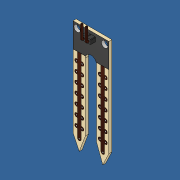
# Autodesk Inventor part: Soil-Moisture-Sensor-Probe
Saved by Autodesk Inventor 2018 (Build 220112000, 112)
## iProperties
Created: 2017-12-22
Part Number: Soil-Moisture-Sensor-Probe
Material: Generisch
Document SubType Name: Modeling
Designer: Martin
Density: 1 g/cm^3
Appearance: Vorgabe
Author: Martin
Autodesk Inventor part; units mm, degrees
ref_plane "YZ Plane" through (0, 0, 0) normal (1, 0, 0) x (0, 1, 0)
sketch "Skizze1" plane through (0, 0, 0) normal (0, 1, 0) x (-1, 0, 0)
  line L0 (9.75, 0) -> (9.75, -53)
  line L1 (9.75, -53) -> (6.4, -60)
  line L2 (6.4, -60) -> (3.05, -51)
  line L3 (3.05, -51) -> (3.05, -14.35)
  arc A0 (3.05, -14.35) -> (-3.05, -14.35) centre (0, -14.35) ccw
  line L4 (-3.05, -14.35) -> (-3.05, -51)
  line L5 (-3.05, -51) -> (-6.4, -60)
  line L6 (-6.4, -60) -> (-9.75, -53)
  line L7 (-9.75, -53) -> (-9.75, 0)
  line L8 (-9.75, 0) -> (9.75, 0)
  line L9 (6.4, -60) -> (-6.4, -60) construction
  line L10 (0, -60) -> (0, -14.35) construction
  circle A1 centre (7.5, -2.5) radius 1.75
  circle A2 centre (-7.5, -2.5) radius 1.75
  line L11 (7.5, -2.5) -> (-7.5, -2.5) construction
  line L12 (0, -2.5) -> (0, -14.35) construction
  point P0 (0, 0)
  point P1 (0, 0)
  dimension "d0" = 19.5
  dimension "d1" = 60
  dimension "d2" = 6.7
  dimension "d3" = 6.7
  dimension "d4" = 11.3
  dimension "d5" = 7
  dimension "d6" = 9
  dimension "d7" = 12.8
  dimension "d8" = 15
  dimension "d9" = 3.5
  dimension "d10" = 0.75
  constraints: 26 end point, 3 centre point, 3 midpoint, 3 parallel, 3 vertical, 2 equal length, 2 horizontal, 2 point on circle, 2 tangent, 1 coincident, 1 equal radius, 1 perpendicular
  measures "d0" distance between parallel lines of L7 L0
  measures "d1" distance from line of L5.end L8
  measures "d2" distance between parallel lines of L7 L4
  measures "d3" distance between parallel lines of L0 L3
  measures "d4" distance edge to line of A0 L8
  measures "d5" vertical distance of L5.end L6.end
  measures "d6" vertical distance of L4.end L5.end
  measures "d7" distance of L1.end L5.end
  measures "d8" distance of L11.start L11.end
  measures "d9" diameter of A2
  measures "d10" distance edge to line of A2 L8
extrude "Extrusion1" add sketch "Skizze1" against normal blind 1.6
sketch "Skizze2" plane through (0, -1.6, 0) normal (0, -1, 0) x (1, 0, 0)
  circle A0 centre (7.5, -2.5) radius 1.75 projected
  circle A1 centre (-7.5, -2.5) radius 1.75 projected
  line L0 (-9.75, 0) -> (-9.75, -53) projected
  line L1 (-9.75, -53) -> (-6.4, -60) projected
  line L2 (-6.4, -60) -> (-3.05, -51) projected
  line L3 (-3.05, -51) -> (-3.05, -14.35) projected
  arc A2 (3.05, -14.35) -> (-3.05, -14.35) centre (0, -14.35) ccw projected
  line L4 (3.05, -14.35) -> (3.05, -51) projected
  line L5 (3.05, -51) -> (6.4, -60) projected
  line L6 (6.4, -60) -> (9.75, -53) projected
  line L7 (9.75, -53) -> (9.75, 0) projected
  line L8 (9.75, 0) -> (-9.75, 0) projected
  line L9 (-7.4, -13.3) -> (-5.4, -13.3)
  line L10 (-5.4, -13.3) -> (-5.4, -54)
  line L11 (-6.4, -55) -> (-6.4, -55)
  line L12 (-7.4, -54) -> (-7.4, -13.3)
  line L13 (5.4, -13.3) -> (7.4, -13.3)
  line L14 (7.4, -13.3) -> (7.4, -54)
  line L15 (6.4, -55) -> (6.4, -55)
  line L16 (5.4, -54) -> (5.4, -13.3)
  arc A3 (5.4, -54) -> (6.4, -55) centre (6.4, -54) ccw
  arc A4 (6.4, -55) -> (7.4, -54) centre (6.4, -54) ccw
  arc A5 (-6.4, -55) -> (-5.4, -54) centre (-6.4, -54) ccw
  arc A6 (-7.4, -54) -> (-6.4, -55) centre (-6.4, -54) ccw
  point P0 (0, 0)
  dimension "d13" = 2
  dimension "d14" = 55
  dimension "d15" = 6.7
  dimension "d16" = 2.35
  dimension "d17" = 2.35
  dimension "d18" = 1
  dimension "d19" = 13.3
  constraints: 16 end point, 8 point on circle, 8 tangent, 4 centre point, 4 parallel, 3 equal radius, 2 collinear, 2 horizontal, 2 perpendicular, 1 point on line
  measures "d13" distance between parallel lines of L14 L16
  measures "d14" distance between parallel lines of L8 L15
  measures "d15" distance between parallel lines of L7 L4
  measures "d16" distance between parallel lines of L7 L14
  measures "d17" distance between parallel lines of L0 L12
  measures "d18" radius of A3
  measures "d19" distance between parallel lines of L8 L13
extrude "Extrusion2" add sketch "Skizze2" along normal blind 0.01 contours L9 L10 A5 A6 L12 | L13 L14 A4 A3 L16
sketch "Skizze3" plane through (0, -1.61, 0) normal (0, -1, 0) x (1, 0, 0)
  line L0 (-5.4, -13.3) -> (-7.4, -13.3) projected
  line L1 (-7.4, -13.3) -> (-7.4, -54) projected
  arc A0 (-7.4, -54) -> (-5.4, -54) centre (-6.4, -54) ccw projected
  line L2 (-5.4, -54) -> (-5.4, -13.3) projected
  line L3 (-8.9, -18) -> (-3.9, -18) construction
  line L4 (-7.9, -19) -> (-4.9, -19)
  line L5 (-4.9, -17) -> (-7.9, -17)
  arc A1 (-7.9, -17) -> (-7.9, -19) centre (-7.9, -18) ccw
  arc A2 (-4.9, -19) -> (-4.9, -17) centre (-4.9, -18) ccw
  line L6 (-6.4, -13.3) -> (-6.4, -54) construction
  line L7 (7.4, -13.3) -> (5.4, -13.3) construction
  arc A3 (-7.9, -22.1) -> (-7.9, -24.1) centre (-7.9, -23.1) ccw
  arc A4 (-4.9, -24.1) -> (-4.9, -22.1) centre (-4.9, -23.1) ccw
  line L8 (-7.9, -24.1) -> (-4.9, -24.1)
  line L9 (-8.9, -23.1) -> (-3.9, -23.1) construction
  line L10 (-4.9, -22.1) -> (-7.9, -22.1)
  arc A5 (-7.9, -27.2) -> (-7.9, -29.2) centre (-7.9, -28.2) ccw
  arc A6 (-4.9, -29.2) -> (-4.9, -27.2) centre (-4.9, -28.2) ccw
  line L11 (-7.9, -29.2) -> (-4.9, -29.2)
  line L12 (-8.9, -28.2) -> (-3.9, -28.2) construction
  line L13 (-4.9, -27.2) -> (-7.9, -27.2)
  arc A7 (-7.9, -32.3) -> (-7.9, -34.3) centre (-7.9, -33.3) ccw
  arc A8 (-4.9, -34.3) -> (-4.9, -32.3) centre (-4.9, -33.3) ccw
  line L14 (-7.9, -34.3) -> (-4.9, -34.3)
  line L15 (-8.9, -33.3) -> (-3.9, -33.3) construction
  line L16 (-4.9, -32.3) -> (-7.9, -32.3)
  arc A9 (-7.9, -37.4) -> (-7.9, -39.4) centre (-7.9, -38.4) ccw
  arc A10 (-4.9, -39.4) -> (-4.9, -37.4) centre (-4.9, -38.4) ccw
  line L17 (-7.9, -39.4) -> (-4.9, -39.4)
  line L18 (-8.9, -38.4) -> (-3.9, -38.4) construction
  line L19 (-4.9, -37.4) -> (-7.9, -37.4)
  arc A11 (-7.9, -42.5) -> (-7.9, -44.5) centre (-7.9, -43.5) ccw
  arc A12 (-4.9, -44.5) -> (-4.9, -42.5) centre (-4.9, -43.5) ccw
  line L20 (-7.9, -44.5) -> (-4.9, -44.5)
  line L21 (-8.9, -43.5) -> (-3.9, -43.5) construction
  line L22 (-4.9, -42.5) -> (-7.9, -42.5)
  arc A13 (-7.9, -47.6) -> (-7.9, -49.6) centre (-7.9, -48.6) ccw
  arc A14 (-4.9, -49.6) -> (-4.9, -47.6) centre (-4.9, -48.6) ccw
  line L23 (-7.9, -49.6) -> (-4.9, -49.6)
  line L24 (-8.9, -48.6) -> (-3.9, -48.6) construction
  line L25 (-4.9, -47.6) -> (-7.9, -47.6)
  arc A15 (4.9, -17) -> (4.9, -19) centre (4.9, -18) ccw
  arc A16 (7.9, -19) -> (7.9, -17) centre (7.9, -18) ccw
  line L26 (4.9, -19) -> (7.9, -19)
  line L27 (3.9, -18) -> (8.9, -18) construction
  line L28 (7.9, -17) -> (4.9, -17)
  arc A17 (4.9, -22.1) -> (4.9, -24.1) centre (4.9, -23.1) ccw
  arc A18 (7.9, -24.1) -> (7.9, -22.1) centre (7.9, -23.1) ccw
  line L29 (4.9, -24.1) -> (7.9, -24.1)
  line L30 (3.9, -23.1) -> (8.9, -23.1) construction
  line L31 (7.9, -22.1) -> (4.9, -22.1)
  arc A19 (4.9, -27.2) -> (4.9, -29.2) centre (4.9, -28.2) ccw
  arc A20 (7.9, -29.2) -> (7.9, -27.2) centre (7.9, -28.2) ccw
  line L32 (4.9, -29.2) -> (7.9, -29.2)
  line L33 (3.9, -28.2) -> (8.9, -28.2) construction
  line L34 (7.9, -27.2) -> (4.9, -27.2)
  arc A21 (4.9, -32.3) -> (4.9, -34.3) centre (4.9, -33.3) ccw
  arc A22 (7.9, -34.3) -> (7.9, -32.3) centre (7.9, -33.3) ccw
  line L35 (4.9, -34.3) -> (7.9, -34.3)
  line L36 (3.9, -33.3) -> (8.9, -33.3) construction
  line L37 (7.9, -32.3) -> (4.9, -32.3)
  arc A23 (4.9, -37.4) -> (4.9, -39.4) centre (4.9, -38.4) ccw
  arc A24 (7.9, -39.4) -> (7.9, -37.4) centre (7.9, -38.4) ccw
  line L38 (4.9, -39.4) -> (7.9, -39.4)
  line L39 (3.9, -38.4) -> (8.9, -38.4) construction
  line L40 (7.9, -37.4) -> (4.9, -37.4)
  arc A25 (4.9, -42.5) -> (4.9, -44.5) centre (4.9, -43.5) ccw
  arc A26 (7.9, -44.5) -> (7.9, -42.5) centre (7.9, -43.5) ccw
  line L41 (4.9, -44.5) -> (7.9, -44.5)
  line L42 (3.9, -43.5) -> (8.9, -43.5) construction
  line L43 (7.9, -42.5) -> (4.9, -42.5)
  arc A27 (4.9, -47.6) -> (4.9, -49.6) centre (4.9, -48.6) ccw
  arc A28 (7.9, -49.6) -> (7.9, -47.6) centre (7.9, -48.6) ccw
  line L44 (4.9, -49.6) -> (7.9, -49.6)
  line L45 (3.9, -48.6) -> (8.9, -48.6) construction
  line L46 (7.9, -47.6) -> (4.9, -47.6)
  point P0 (0, 0)
  point P1 (-6.4, -18)
  point P2 (-6.4, -23.1)
  point P3 (-6.4, -28.2)
  point P4 (-6.4, -33.3)
  point P5 (-6.4, -38.4)
  point P6 (-6.4, -43.5)
  point P7 (-6.4, -48.6)
  point P8 (6.4, -18)
  point P9 (6.4, -23.1)
  point P10 (6.4, -28.2)
  point P11 (6.4, -33.3)
  point P12 (6.4, -38.4)
  point P13 (6.4, -43.5)
  point P14 (6.4, -48.6)
  dimension "d22" = 18
  dimension "d23" = 12.8
  dimension "d24" = 3
  dimension "d25" = 2
  dimension "d28" = 5.1
  dimension "d31" = 12.8
  constraints: 114 end point, 84 point on circle, 29 point on line, 28 centre point, 4 tangent, 2 midpoint, 2 vertical, 1 horizontal, 1 parallel, 1 perpendicular, 182 other
  measures "d22" distance from line of point (0, 0) L3
  measures "d23" distance of L7.end L0.end
  measures "d24" distance of A1.centre A2.centre
  measures "d25" distance between parallel lines of L5 L4
  measures "d28" distance of A1.centre A3.centre
  measures "d31" distance of A1.centre A15.centre
extrude "Extrusion3" add sketch "Skizze3" against normal blind 0.01 contours L5 A2 L4 L2 | L2 L4 L1 L5 | L1 L4 A1 L5 | L10 A4 L8 L2 | L2 L8 L1 L10 | L1 L8 A3 L10 | L13 A6 L11 L2 | L2 L11 L1 L13 | L1 L11 A5 L13 | L16 A8 L14 L2 | L2 L14 L1 L16 | L1 L14 A7 L16 | L19 A10 L17 L2 | L2 L17 L1 L19 | L1 L17 A9 L19 | L22 A12 L20 L2 | L2 L20 L1 L22 | L1 L20 A11 L22 | L25 A14 L23 L2 | L2 L23 L1 L25 | L1 L23 A13 L25 | L28 A16 L26 A15 | L31 A18 L29 A17 | L34 A20 L32 A19 | L37 A22 L35 A21 | L40 A24 L38 A23 | L43 A26 L41 A25 | L46 A28 L44 A27
ref_plane "Arbeitsebene1" through (0, -0.8, 0) normal (0, -1, 0) x (1, 0, 0)
sketch "Skizze4" plane through (0, -1.6, 0) normal (0, -1, 0) x (1, 0, 0)
  line L0 (-4.9, -49.6) -> (-5.4, -49.6) projected
  line L1 (-5.4, -49.6) -> (-5.4, -54) projected
  arc A0 (-7.4, -54) -> (-5.4, -54) centre (-6.4, -54) ccw projected
  line L2 (-7.4, -54) -> (-7.4, -49.6) projected
  line L3 (-7.4, -49.6) -> (-7.9, -49.6) projected
  arc A1 (-7.9, -47.6) -> (-7.9, -49.6) centre (-7.9, -48.6) ccw projected
  line L4 (-7.9, -47.6) -> (-7.4, -47.6) projected
  line L5 (-7.4, -47.6) -> (-7.4, -44.5) projected
  line L6 (-7.4, -44.5) -> (-7.9, -44.5) projected
  arc A2 (-7.9, -42.5) -> (-7.9, -44.5) centre (-7.9, -43.5) ccw projected
  line L7 (-7.9, -42.5) -> (-7.4, -42.5) projected
  line L8 (-7.4, -42.5) -> (-7.4, -39.4) projected
  line L9 (-7.4, -39.4) -> (-7.9, -39.4) projected
  arc A3 (-7.9, -37.4) -> (-7.9, -39.4) centre (-7.9, -38.4) ccw projected
  line L10 (-7.9, -37.4) -> (-7.4, -37.4) projected
  line L11 (-7.4, -37.4) -> (-7.4, -34.3) projected
  line L12 (-7.4, -34.3) -> (-7.9, -34.3) projected
  arc A4 (-7.9, -32.3) -> (-7.9, -34.3) centre (-7.9, -33.3) ccw projected
  line L13 (-7.9, -32.3) -> (-7.4, -32.3) projected
  line L14 (-7.4, -32.3) -> (-7.4, -29.2) projected
  line L15 (-7.4, -29.2) -> (-7.9, -29.2) projected
  arc A5 (-7.9, -27.2) -> (-7.9, -29.2) centre (-7.9, -28.2) ccw projected
  line L16 (-7.9, -27.2) -> (-7.4, -27.2) projected
  line L17 (-7.4, -27.2) -> (-7.4, -24.1) projected
  line L18 (-7.4, -24.1) -> (-7.9, -24.1) projected
  arc A6 (-7.9, -22.1) -> (-7.9, -24.1) centre (-7.9, -23.1) ccw projected
  line L19 (-7.9, -22.1) -> (-7.4, -22.1) projected
  line L20 (-7.4, -22.1) -> (-7.4, -19) projected
  line L21 (-7.4, -19) -> (-7.9, -19) projected
  arc A7 (-7.9, -17) -> (-7.9, -19) centre (-7.9, -18) ccw projected
  line L22 (-7.9, -17) -> (-7.4, -17) projected
  line L23 (-7.4, -17) -> (-7.4, -13.3) projected
  line L24 (-7.4, -13.3) -> (-5.4, -13.3) projected
  line L25 (-5.4, -13.3) -> (-5.4, -17) projected
  line L26 (-5.4, -17) -> (-4.9, -17) projected
  arc A8 (-4.9, -19) -> (-4.9, -17) centre (-4.9, -18) ccw projected
  line L27 (-4.9, -19) -> (-5.4, -19) projected
  line L28 (-5.4, -19) -> (-5.4, -22.1) projected
  line L29 (-5.4, -22.1) -> (-4.9, -22.1) projected
  arc A9 (-4.9, -24.1) -> (-4.9, -22.1) centre (-4.9, -23.1) ccw projected
  line L30 (-4.9, -24.1) -> (-5.4, -24.1) projected
  line L31 (-5.4, -24.1) -> (-5.4, -27.2) projected
  line L32 (-5.4, -27.2) -> (-4.9, -27.2) projected
  arc A10 (-4.9, -29.2) -> (-4.9, -27.2) centre (-4.9, -28.2) ccw projected
  line L33 (-4.9, -29.2) -> (-5.4, -29.2) projected
  line L34 (-5.4, -29.2) -> (-5.4, -32.3) projected
  line L35 (-5.4, -32.3) -> (-4.9, -32.3) projected
  arc A11 (-4.9, -34.3) -> (-4.9, -32.3) centre (-4.9, -33.3) ccw projected
  line L36 (-4.9, -34.3) -> (-5.4, -34.3) projected
  line L37 (-5.4, -34.3) -> (-5.4, -37.4) projected
  line L38 (-5.4, -37.4) -> (-4.9, -37.4) projected
  arc A12 (-4.9, -39.4) -> (-4.9, -37.4) centre (-4.9, -38.4) ccw projected
  line L39 (-4.9, -39.4) -> (-5.4, -39.4) projected
  line L40 (-5.4, -39.4) -> (-5.4, -42.5) projected
  line L41 (-5.4, -42.5) -> (-4.9, -42.5) projected
  arc A13 (-4.9, -44.5) -> (-4.9, -42.5) centre (-4.9, -43.5) ccw projected
  line L42 (-4.9, -44.5) -> (-5.4, -44.5) projected
  line L43 (-5.4, -44.5) -> (-5.4, -47.6) projected
  line L44 (-5.4, -47.6) -> (-4.9, -47.6) projected
  arc A14 (-4.9, -49.6) -> (-4.9, -47.6) centre (-4.9, -48.6) ccw projected
  line L45 (7.9, -44.5) -> (7.4, -44.5) projected
  line L46 (7.4, -44.5) -> (7.4, -47.6) projected
  line L47 (7.4, -47.6) -> (7.9, -47.6) projected
  arc A15 (7.9, -49.6) -> (7.9, -47.6) centre (7.9, -48.6) ccw projected
  line L48 (7.9, -49.6) -> (7.4, -49.6) projected
  line L49 (7.4, -49.6) -> (7.4, -54) projected
  arc A16 (5.4, -54) -> (7.4, -54) centre (6.4, -54) ccw projected
  line L50 (5.4, -54) -> (5.4, -49.6) projected
  line L51 (5.4, -49.6) -> (4.9, -49.6) projected
  arc A17 (4.9, -47.6) -> (4.9, -49.6) centre (4.9, -48.6) ccw projected
  line L52 (4.9, -47.6) -> (5.4, -47.6) projected
  line L53 (5.4, -47.6) -> (5.4, -44.5) projected
  line L54 (5.4, -44.5) -> (4.9, -44.5) projected
  arc A18 (4.9, -42.5) -> (4.9, -44.5) centre (4.9, -43.5) ccw projected
  line L55 (4.9, -42.5) -> (5.4, -42.5) projected
  line L56 (5.4, -42.5) -> (5.4, -39.4) projected
  line L57 (5.4, -39.4) -> (4.9, -39.4) projected
  arc A19 (4.9, -37.4) -> (4.9, -39.4) centre (4.9, -38.4) ccw projected
  line L58 (4.9, -37.4) -> (5.4, -37.4) projected
  line L59 (5.4, -37.4) -> (5.4, -34.3) projected
  line L60 (5.4, -34.3) -> (4.9, -34.3) projected
  arc A20 (4.9, -32.3) -> (4.9, -34.3) centre (4.9, -33.3) ccw projected
  line L61 (4.9, -32.3) -> (5.4, -32.3) projected
  line L62 (5.4, -32.3) -> (5.4, -29.2) projected
  line L63 (5.4, -29.2) -> (4.9, -29.2) projected
  arc A21 (4.9, -27.2) -> (4.9, -29.2) centre (4.9, -28.2) ccw projected
  line L64 (4.9, -27.2) -> (5.4, -27.2) projected
  line L65 (5.4, -27.2) -> (5.4, -24.1) projected
  line L66 (5.4, -24.1) -> (4.9, -24.1) projected
  arc A22 (4.9, -22.1) -> (4.9, -24.1) centre (4.9, -23.1) ccw projected
  line L67 (4.9, -22.1) -> (5.4, -22.1) projected
  line L68 (5.4, -22.1) -> (5.4, -19) projected
  line L69 (5.4, -19) -> (4.9, -19) projected
  arc A23 (4.9, -17) -> (4.9, -19) centre (4.9, -18) ccw projected
  line L70 (4.9, -17) -> (5.4, -17) projected
  line L71 (5.4, -17) -> (5.4, -13.3) projected
  line L72 (5.4, -13.3) -> (7.4, -13.3) projected
  line L73 (7.4, -13.3) -> (7.4, -17) projected
  line L74 (7.4, -17) -> (7.9, -17) projected
  arc A24 (7.9, -19) -> (7.9, -17) centre (7.9, -18) ccw projected
  line L75 (7.9, -19) -> (7.4, -19) projected
  line L76 (7.4, -19) -> (7.4, -22.1) projected
  line L77 (7.4, -22.1) -> (7.9, -22.1) projected
  arc A25 (7.9, -24.1) -> (7.9, -22.1) centre (7.9, -23.1) ccw projected
  line L78 (7.9, -24.1) -> (7.4, -24.1) projected
  line L79 (7.4, -24.1) -> (7.4, -27.2) projected
  line L80 (7.4, -27.2) -> (7.9, -27.2) projected
  arc A26 (7.9, -29.2) -> (7.9, -27.2) centre (7.9, -28.2) ccw projected
  line L81 (7.9, -29.2) -> (7.4, -29.2) projected
  line L82 (7.4, -29.2) -> (7.4, -32.3) projected
  line L83 (7.4, -32.3) -> (7.9, -32.3) projected
  arc A27 (7.9, -34.3) -> (7.9, -32.3) centre (7.9, -33.3) ccw projected
  line L84 (7.9, -34.3) -> (7.4, -34.3) projected
  line L85 (7.4, -34.3) -> (7.4, -37.4) projected
  line L86 (7.4, -37.4) -> (7.9, -37.4) projected
  arc A28 (7.9, -39.4) -> (7.9, -37.4) centre (7.9, -38.4) ccw projected
  line L87 (7.9, -39.4) -> (7.4, -39.4) projected
  line L88 (7.4, -39.4) -> (7.4, -42.5) projected
  line L89 (7.4, -42.5) -> (7.9, -42.5) projected
  arc A29 (7.9, -44.5) -> (7.9, -42.5) centre (7.9, -43.5) ccw projected
  circle A30 centre (7.5, -2.5) radius 1.75 projected
  circle A31 centre (-7.5, -2.5) radius 1.75 projected
  line L90 (-9.75, 0) -> (-9.75, -53) projected
  line L91 (-9.75, -53) -> (-6.4, -60) projected
  line L92 (-6.4, -60) -> (-3.05, -51) projected
  line L93 (-3.05, -51) -> (-3.05, -14.35) projected
  arc A32 (3.05, -14.35) -> (-3.05, -14.35) centre (0, -14.35) ccw projected
  line L94 (3.05, -14.35) -> (3.05, -51) projected
  line L95 (3.05, -51) -> (6.4, -60) projected
  line L96 (6.4, -60) -> (9.75, -53) projected
  line L97 (9.75, -53) -> (9.75, 0) projected
  line L98 (9.75, 0) -> (-9.75, 0) projected
  line L99 (-7.4, -49.6) -> (-7.4, -54) projected
  arc A33 (-7.4, -54) -> (-5.4, -54) centre (-6.4, -54) ccw projected
  line L100 (-5.4, -54) -> (-5.4, -49.6) projected
  line L101 (-4.9, -49.6) -> (-5.4, -49.6) projected
  arc A34 (-4.9, -49.6) -> (-4.9, -47.6) centre (-4.9, -48.6) ccw projected
  line L102 (-5.4, -47.6) -> (-4.9, -47.6) projected
  line L103 (-5.4, -47.6) -> (-5.4, -44.5) projected
  line L104 (-4.9, -44.5) -> (-5.4, -44.5) projected
  arc A35 (-4.9, -44.5) -> (-4.9, -42.5) centre (-4.9, -43.5) ccw projected
  line L105 (-5.4, -42.5) -> (-4.9, -42.5) projected
  line L106 (-5.4, -42.5) -> (-5.4, -39.4) projected
  line L107 (-4.9, -39.4) -> (-5.4, -39.4) projected
  arc A36 (-4.9, -39.4) -> (-4.9, -37.4) centre (-4.9, -38.4) ccw projected
  line L108 (-5.4, -37.4) -> (-4.9, -37.4) projected
  line L109 (-5.4, -37.4) -> (-5.4, -34.3) projected
  line L110 (-4.9, -34.3) -> (-5.4, -34.3) projected
  arc A37 (-4.9, -34.3) -> (-4.9, -32.3) centre (-4.9, -33.3) ccw projected
  line L111 (-5.4, -32.3) -> (-4.9, -32.3) projected
  line L112 (-5.4, -32.3) -> (-5.4, -29.2) projected
  line L113 (-4.9, -29.2) -> (-5.4, -29.2) projected
  arc A38 (-4.9, -29.2) -> (-4.9, -27.2) centre (-4.9, -28.2) ccw projected
  line L114 (-5.4, -27.2) -> (-4.9, -27.2) projected
  line L115 (-5.4, -27.2) -> (-5.4, -24.1) projected
  line L116 (-4.9, -24.1) -> (-5.4, -24.1) projected
  arc A39 (-4.9, -24.1) -> (-4.9, -22.1) centre (-4.9, -23.1) ccw projected
  line L117 (-5.4, -22.1) -> (-4.9, -22.1) projected
  line L118 (-5.4, -22.1) -> (-5.4, -19) projected
  line L119 (-5.4, -19) -> (-4.9, -19) projected
  arc A40 (-4.9, -19) -> (-4.9, -17) centre (-4.9, -18) ccw projected
  line L120 (-4.9, -17) -> (-5.4, -17) projected
  line L121 (-5.4, -17) -> (-5.4, -13.3) projected
  line L122 (-5.4, -13.3) -> (-7.4, -13.3) projected
  line L123 (-7.4, -13.3) -> (-7.4, -17) projected
  line L124 (-7.4, -17) -> (-7.9, -17) projected
  arc A41 (-7.9, -17) -> (-7.9, -19) centre (-7.9, -18) ccw projected
  line L125 (-7.9, -19) -> (-7.4, -19) projected
  line L126 (-7.4, -19) -> (-7.4, -22.1) projected
  line L127 (-7.9, -22.1) -> (-7.4, -22.1) projected
  arc A42 (-7.9, -22.1) -> (-7.9, -24.1) centre (-7.9, -23.1) ccw projected
  line L128 (-7.4, -24.1) -> (-7.9, -24.1) projected
  line L129 (-7.4, -24.1) -> (-7.4, -27.2) projected
  line L130 (-7.9, -27.2) -> (-7.4, -27.2) projected
  arc A43 (-7.9, -27.2) -> (-7.9, -29.2) centre (-7.9, -28.2) ccw projected
  line L131 (-7.4, -29.2) -> (-7.9, -29.2) projected
  line L132 (-7.4, -29.2) -> (-7.4, -32.3) projected
  line L133 (-7.9, -32.3) -> (-7.4, -32.3) projected
  arc A44 (-7.9, -32.3) -> (-7.9, -34.3) centre (-7.9, -33.3) ccw projected
  line L134 (-7.4, -34.3) -> (-7.9, -34.3) projected
  line L135 (-7.4, -34.3) -> (-7.4, -37.4) projected
  line L136 (-7.9, -37.4) -> (-7.4, -37.4) projected
  arc A45 (-7.9, -37.4) -> (-7.9, -39.4) centre (-7.9, -38.4) ccw projected
  line L137 (-7.4, -39.4) -> (-7.9, -39.4) projected
  line L138 (-7.4, -39.4) -> (-7.4, -42.5) projected
  line L139 (-7.9, -42.5) -> (-7.4, -42.5) projected
  arc A46 (-7.9, -42.5) -> (-7.9, -44.5) centre (-7.9, -43.5) ccw projected
  line L140 (-7.4, -44.5) -> (-7.9, -44.5) projected
  line L141 (-7.4, -44.5) -> (-7.4, -47.6) projected
  line L142 (-7.9, -47.6) -> (-7.4, -47.6) projected
  arc A47 (-7.9, -47.6) -> (-7.9, -49.6) centre (-7.9, -48.6) ccw projected
  line L143 (-7.4, -49.6) -> (-7.9, -49.6) projected
  line L144 (5.4, -49.6) -> (5.4, -54) projected
  arc A48 (5.4, -54) -> (7.4, -54) centre (6.4, -54) ccw projected
  line L145 (7.4, -54) -> (7.4, -49.6) projected
  line L146 (7.9, -49.6) -> (7.4, -49.6) projected
  arc A49 (7.9, -49.6) -> (7.9, -47.6) centre (7.9, -48.6) ccw projected
  line L147 (7.4, -47.6) -> (7.9, -47.6) projected
  line L148 (7.4, -47.6) -> (7.4, -44.5) projected
  line L149 (7.9, -44.5) -> (7.4, -44.5) projected
  arc A50 (7.9, -44.5) -> (7.9, -42.5) centre (7.9, -43.5) ccw projected
  line L150 (7.4, -42.5) -> (7.9, -42.5) projected
  line L151 (7.4, -42.5) -> (7.4, -39.4) projected
  line L152 (7.9, -39.4) -> (7.4, -39.4) projected
  arc A51 (7.9, -39.4) -> (7.9, -37.4) centre (7.9, -38.4) ccw projected
  line L153 (7.4, -37.4) -> (7.9, -37.4) projected
  line L154 (7.4, -37.4) -> (7.4, -34.3) projected
  line L155 (7.9, -34.3) -> (7.4, -34.3) projected
  arc A52 (7.9, -34.3) -> (7.9, -32.3) centre (7.9, -33.3) ccw projected
  line L156 (7.4, -32.3) -> (7.9, -32.3) projected
  line L157 (7.4, -32.3) -> (7.4, -29.2) projected
  line L158 (7.9, -29.2) -> (7.4, -29.2) projected
  arc A53 (7.9, -29.2) -> (7.9, -27.2) centre (7.9, -28.2) ccw projected
  line L159 (7.4, -27.2) -> (7.9, -27.2) projected
  line L160 (7.4, -27.2) -> (7.4, -24.1) projected
  line L161 (7.9, -24.1) -> (7.4, -24.1) projected
  arc A54 (7.9, -24.1) -> (7.9, -22.1) centre (7.9, -23.1) ccw projected
  line L162 (7.4, -22.1) -> (7.9, -22.1) projected
  line L163 (7.4, -22.1) -> (7.4, -19) projected
  line L164 (7.9, -19) -> (7.4, -19) projected
  arc A55 (7.9, -19) -> (7.9, -17) centre (7.9, -18) ccw projected
  line L165 (7.4, -17) -> (7.9, -17) projected
  line L166 (7.4, -17) -> (7.4, -13.3) projected
  line L167 (7.4, -13.3) -> (5.4, -13.3) projected
  line L168 (5.4, -13.3) -> (5.4, -17) projected
  line L169 (4.9, -17) -> (5.4, -17) projected
  arc A56 (4.9, -17) -> (4.9, -19) centre (4.9, -18) ccw projected
  line L170 (5.4, -19) -> (4.9, -19) projected
  line L171 (5.4, -19) -> (5.4, -22.1) projected
  line L172 (4.9, -22.1) -> (5.4, -22.1) projected
  arc A57 (4.9, -22.1) -> (4.9, -24.1) centre (4.9, -23.1) ccw projected
  line L173 (5.4, -24.1) -> (4.9, -24.1) projected
  line L174 (5.4, -24.1) -> (5.4, -27.2) projected
  line L175 (4.9, -27.2) -> (5.4, -27.2) projected
  arc A58 (4.9, -27.2) -> (4.9, -29.2) centre (4.9, -28.2) ccw projected
  line L176 (5.4, -29.2) -> (4.9, -29.2) projected
  line L177 (5.4, -29.2) -> (5.4, -32.3) projected
  line L178 (4.9, -32.3) -> (5.4, -32.3) projected
  arc A59 (4.9, -32.3) -> (4.9, -34.3) centre (4.9, -33.3) ccw projected
  line L179 (5.4, -34.3) -> (4.9, -34.3) projected
  line L180 (5.4, -34.3) -> (5.4, -37.4) projected
  line L181 (4.9, -37.4) -> (5.4, -37.4) projected
  arc A60 (4.9, -37.4) -> (4.9, -39.4) centre (4.9, -38.4) ccw projected
  line L182 (5.4, -39.4) -> (4.9, -39.4) projected
  line L183 (5.4, -39.4) -> (5.4, -42.5) projected
  line L184 (4.9, -42.5) -> (5.4, -42.5) projected
  arc A61 (4.9, -42.5) -> (4.9, -44.5) centre (4.9, -43.5) ccw projected
  line L185 (5.4, -44.5) -> (4.9, -44.5) projected
  line L186 (5.4, -44.5) -> (5.4, -47.6) projected
  line L187 (4.9, -47.6) -> (5.4, -47.6) projected
  arc A62 (4.9, -47.6) -> (4.9, -49.6) centre (4.9, -48.6) ccw projected
  line L188 (5.4, -49.6) -> (4.9, -49.6) projected
  line L189 (-7.4, -13.3) -> (-9.75, -13.3)
  line L190 (-5.4, -13.3) -> (-2.8636, -13.3)
  line L191 (5.4, -13.3) -> (2.8636, -13.3)
  line L192 (7.4, -13.3) -> (9.75, -13.3)
  point P0 (0, 0)
  constraints: 8 end point, 5 point on line, 2 point on circle, 1 perpendicular
extrude "Extrusion4" add sketch "Skizze4" along normal blind 0.05 contours L24 L189 L90 L98 L97 L192 L72 L191 A32 L190
mirror "Spiegeln1" about plane through (0, -0.8, 0) normal (0, -1, 0) of "Extrusion2", "Extrusion3", "Extrusion4"
sketch "Skizze5" plane through (0, -1.61, 0) normal (0, -1, 0) x (1, 0, 0)
  line L0 (-7.4, -49.6) -> (-7.4, -54) projected
  arc A0 (-7.4, -54) -> (-5.4, -54) centre (-6.4, -54) ccw projected
  line L1 (-5.4, -54) -> (-5.4, -49.6) projected
  line L2 (-4.9, -49.6) -> (-5.4, -49.6) projected
  arc A1 (-4.9, -49.6) -> (-4.9, -47.6) centre (-4.9, -48.6) ccw projected
  line L3 (-5.4, -47.6) -> (-4.9, -47.6) projected
  line L4 (-5.4, -47.6) -> (-5.4, -44.5) projected
  line L5 (-4.9, -44.5) -> (-5.4, -44.5) projected
  arc A2 (-4.9, -44.5) -> (-4.9, -42.5) centre (-4.9, -43.5) ccw projected
  line L6 (-5.4, -42.5) -> (-4.9, -42.5) projected
  line L7 (-5.4, -42.5) -> (-5.4, -39.4) projected
  line L8 (-4.9, -39.4) -> (-5.4, -39.4) projected
  arc A3 (-4.9, -39.4) -> (-4.9, -37.4) centre (-4.9, -38.4) ccw projected
  line L9 (-5.4, -37.4) -> (-4.9, -37.4) projected
  line L10 (-5.4, -37.4) -> (-5.4, -34.3) projected
  line L11 (-4.9, -34.3) -> (-5.4, -34.3) projected
  arc A4 (-4.9, -34.3) -> (-4.9, -32.3) centre (-4.9, -33.3) ccw projected
  line L12 (-5.4, -32.3) -> (-4.9, -32.3) projected
  line L13 (-5.4, -32.3) -> (-5.4, -29.2) projected
  line L14 (-4.9, -29.2) -> (-5.4, -29.2) projected
  arc A5 (-4.9, -29.2) -> (-4.9, -27.2) centre (-4.9, -28.2) ccw projected
  line L15 (-5.4, -27.2) -> (-4.9, -27.2) projected
  line L16 (-5.4, -27.2) -> (-5.4, -24.1) projected
  line L17 (-4.9, -24.1) -> (-5.4, -24.1) projected
  arc A6 (-4.9, -24.1) -> (-4.9, -22.1) centre (-4.9, -23.1) ccw projected
  line L18 (-5.4, -22.1) -> (-4.9, -22.1) projected
  line L19 (-5.4, -22.1) -> (-5.4, -19) projected
  line L20 (-5.4, -19) -> (-4.9, -19) projected
  arc A7 (-4.9, -19) -> (-4.9, -17) centre (-4.9, -18) ccw projected
  line L21 (-4.9, -17) -> (-5.4, -17) projected
  line L22 (-5.4, -17) -> (-5.4, -13.3) projected
  line L23 (-5.4, -13.3) -> (-7.4, -13.3) projected
  line L24 (-7.4, -13.3) -> (-7.4, -17) projected
  line L25 (-7.4, -17) -> (-7.9, -17) projected
  arc A8 (-7.9, -17) -> (-7.9, -19) centre (-7.9, -18) ccw projected
  line L26 (-7.9, -19) -> (-7.4, -19) projected
  line L27 (-7.4, -19) -> (-7.4, -22.1) projected
  line L28 (-7.9, -22.1) -> (-7.4, -22.1) projected
  arc A9 (-7.9, -22.1) -> (-7.9, -24.1) centre (-7.9, -23.1) ccw projected
  line L29 (-7.4, -24.1) -> (-7.9, -24.1) projected
  line L30 (-7.4, -24.1) -> (-7.4, -27.2) projected
  line L31 (-7.9, -27.2) -> (-7.4, -27.2) projected
  arc A10 (-7.9, -27.2) -> (-7.9, -29.2) centre (-7.9, -28.2) ccw projected
  line L32 (-7.4, -29.2) -> (-7.9, -29.2) projected
  line L33 (-7.4, -29.2) -> (-7.4, -32.3) projected
  line L34 (-7.9, -32.3) -> (-7.4, -32.3) projected
  arc A11 (-7.9, -32.3) -> (-7.9, -34.3) centre (-7.9, -33.3) ccw projected
  line L35 (-7.4, -34.3) -> (-7.9, -34.3) projected
  line L36 (-7.4, -34.3) -> (-7.4, -37.4) projected
  line L37 (-7.9, -37.4) -> (-7.4, -37.4) projected
  arc A12 (-7.9, -37.4) -> (-7.9, -39.4) centre (-7.9, -38.4) ccw projected
  line L38 (-7.4, -39.4) -> (-7.9, -39.4) projected
  line L39 (-7.4, -39.4) -> (-7.4, -42.5) projected
  line L40 (-7.9, -42.5) -> (-7.4, -42.5) projected
  arc A13 (-7.9, -42.5) -> (-7.9, -44.5) centre (-7.9, -43.5) ccw projected
  line L41 (-7.4, -44.5) -> (-7.9, -44.5) projected
  line L42 (-7.4, -44.5) -> (-7.4, -47.6) projected
  line L43 (-7.9, -47.6) -> (-7.4, -47.6) projected
  arc A14 (-7.9, -47.6) -> (-7.9, -49.6) centre (-7.9, -48.6) ccw projected
  line L44 (-7.4, -49.6) -> (-7.9, -49.6) projected
  line L45 (5.4, -49.6) -> (5.4, -54) projected
  arc A15 (5.4, -54) -> (7.4, -54) centre (6.4, -54) ccw projected
  line L46 (7.4, -54) -> (7.4, -49.6) projected
  line L47 (7.9, -49.6) -> (7.4, -49.6) projected
  arc A16 (7.9, -49.6) -> (7.9, -47.6) centre (7.9, -48.6) ccw projected
  line L48 (7.4, -47.6) -> (7.9, -47.6) projected
  line L49 (7.4, -47.6) -> (7.4, -44.5) projected
  line L50 (7.9, -44.5) -> (7.4, -44.5) projected
  arc A17 (7.9, -44.5) -> (7.9, -42.5) centre (7.9, -43.5) ccw projected
  line L51 (7.4, -42.5) -> (7.9, -42.5) projected
  line L52 (7.4, -42.5) -> (7.4, -39.4) projected
  line L53 (7.9, -39.4) -> (7.4, -39.4) projected
  arc A18 (7.9, -39.4) -> (7.9, -37.4) centre (7.9, -38.4) ccw projected
  line L54 (7.4, -37.4) -> (7.9, -37.4) projected
  line L55 (7.4, -37.4) -> (7.4, -34.3) projected
  line L56 (7.9, -34.3) -> (7.4, -34.3) projected
  arc A19 (7.9, -34.3) -> (7.9, -32.3) centre (7.9, -33.3) ccw projected
  line L57 (7.4, -32.3) -> (7.9, -32.3) projected
  line L58 (7.4, -32.3) -> (7.4, -29.2) projected
  line L59 (7.9, -29.2) -> (7.4, -29.2) projected
  arc A20 (7.9, -29.2) -> (7.9, -27.2) centre (7.9, -28.2) ccw projected
  line L60 (7.4, -27.2) -> (7.9, -27.2) projected
  line L61 (7.4, -27.2) -> (7.4, -24.1) projected
  line L62 (7.9, -24.1) -> (7.4, -24.1) projected
  arc A21 (7.9, -24.1) -> (7.9, -22.1) centre (7.9, -23.1) ccw projected
  line L63 (7.4, -22.1) -> (7.9, -22.1) projected
  line L64 (7.4, -22.1) -> (7.4, -19) projected
  line L65 (7.9, -19) -> (7.4, -19) projected
  arc A22 (7.9, -19) -> (7.9, -17) centre (7.9, -18) ccw projected
  line L66 (7.4, -17) -> (7.9, -17) projected
  line L67 (7.4, -17) -> (7.4, -13.3) projected
  line L68 (7.4, -13.3) -> (5.4, -13.3) projected
  line L69 (5.4, -13.3) -> (5.4, -17) projected
  line L70 (4.9, -17) -> (5.4, -17) projected
  arc A23 (4.9, -17) -> (4.9, -19) centre (4.9, -18) ccw projected
  line L71 (5.4, -19) -> (4.9, -19) projected
  line L72 (5.4, -19) -> (5.4, -22.1) projected
  line L73 (4.9, -22.1) -> (5.4, -22.1) projected
  arc A24 (4.9, -22.1) -> (4.9, -24.1) centre (4.9, -23.1) ccw projected
  line L74 (5.4, -24.1) -> (4.9, -24.1) projected
  line L75 (5.4, -24.1) -> (5.4, -27.2) projected
  line L76 (4.9, -27.2) -> (5.4, -27.2) projected
  arc A25 (4.9, -27.2) -> (4.9, -29.2) centre (4.9, -28.2) ccw projected
  line L77 (5.4, -29.2) -> (4.9, -29.2) projected
  line L78 (5.4, -29.2) -> (5.4, -32.3) projected
  line L79 (4.9, -32.3) -> (5.4, -32.3) projected
  arc A26 (4.9, -32.3) -> (4.9, -34.3) centre (4.9, -33.3) ccw projected
  line L80 (5.4, -34.3) -> (4.9, -34.3) projected
  line L81 (5.4, -34.3) -> (5.4, -37.4) projected
  line L82 (4.9, -37.4) -> (5.4, -37.4) projected
  arc A27 (4.9, -37.4) -> (4.9, -39.4) centre (4.9, -38.4) ccw projected
  line L83 (5.4, -39.4) -> (4.9, -39.4) projected
  line L84 (5.4, -39.4) -> (5.4, -42.5) projected
  line L85 (4.9, -42.5) -> (5.4, -42.5) projected
  arc A28 (4.9, -42.5) -> (4.9, -44.5) centre (4.9, -43.5) ccw projected
  line L86 (5.4, -44.5) -> (4.9, -44.5) projected
  line L87 (5.4, -44.5) -> (5.4, -47.6) projected
  line L88 (4.9, -47.6) -> (5.4, -47.6) projected
  arc A29 (4.9, -47.6) -> (4.9, -49.6) centre (4.9, -48.6) ccw projected
  line L89 (5.4, -49.6) -> (4.9, -49.6) projected
  point P0 (0, 0)
hole "Bohrung1" at (-7.9, -1.61, -18) at (-4.9, -1.61, -18) at (4.9, -1.61, -18) at (7.9, -1.61, -18) at (-7.9, -1.61, -23.1) at (-4.9, -1.61, -23.1) at (4.9, -1.61, -23.1) at (7.9, -1.61, -23.1) at (-7.9, -1.61, -28.2) at (-4.9, -1.61, -28.2) at (4.9, -1.61, -28.2) at (7.9, -1.61, -28.2) at (-7.9, -1.61, -33.3) at (-4.9, -1.61, -33.3) at (4.9, -1.61, -33.3) at (7.9, -1.61, -33.3) at (-7.9, -1.61, -38.4) at (-4.9, -1.61, -38.4) at (4.9, -1.61, -38.4) at (7.9, -1.61, -38.4) at (-7.9, -1.61, -43.5) at (-4.9, -1.61, -43.5) at (4.9, -1.61, -43.5) at (7.9, -1.61, -43.5) at (-7.9, -1.61, -48.6) at (-4.9, -1.61, -48.6) at (4.9, -1.61, -48.6) at (7.9, -1.61, -48.6) at (-6.4, -1.61, -54) at (6.4, -1.61, -54) direction (0, 1, 0) diameter 0.8 end through all
sketch "Skizze6" plane through (0, -1.65, 0) normal (0, -1, 0) x (1, 0, 0)
  line L0 (-2.54, -1.5) -> (0, -1.5)
  line L1 (0, -1.5) -> (0, -4.04)
  line L2 (0, -4.04) -> (-2.54, -4.04)
  line L3 (-2.54, -4.04) -> (-2.54, -1.5)
  point P0 (0, 0)
  dimension "d45" = 2.54
  dimension "d46" = 1.5
  constraints: 8 end point, 2 parallel, 2 perpendicular, 1 horizontal, 1 point on line
  measures "d45" distance of L0.start L0.end
  measures "d46" distance from line of point (0, 0) L0
extrude "Extrusion5" add sketch "Skizze6" along normal blind 2.54
chamfer "Fase1" distance 0.254 angle 45 4 edges at (-2.54, -2.92, -1.5) (0, -2.92, -1.5) (0, -2.92, -4.04) (-2.54, -2.92, -4.04)
ref_plane "Arbeitsebene2" through (0, 1.35, 0) normal (0, -1, 0) x (1, 0, 0)
sketch "Skizze7" plane through (0, 1.35, 0) normal (0, -1, 0) x (1, 0, 0)
  line L0 (-2.286, -4.04) -> (-2.54, -3.786) projected
  line L1 (-2.286, -4.04) -> (-0.254, -4.04) projected
  line L2 (0, -3.786) -> (-0.254, -4.04) projected
  line L3 (0, -3.786) -> (0, -1.754) projected
  line L4 (-0.254, -1.5) -> (0, -1.754) projected
  line L5 (-0.254, -1.5) -> (-2.286, -1.5) projected
  line L6 (-2.54, -1.754) -> (-2.286, -1.5) projected
  line L7 (-2.54, -1.754) -> (-2.54, -3.786) projected
  line L8 (-1.62, -2.42) -> (-0.92, -2.42)
  line L9 (-0.92, -2.42) -> (-0.92, -3.12)
  line L10 (-0.92, -3.12) -> (-1.62, -3.12)
  line L11 (-1.62, -3.12) -> (-1.62, -2.42)
  point P0 (0, 0)
  dimension "d53" = 0.7
  constraints: 8 end point, 3 other
  measures "d53" distance of L8.start L8.end
extrude "Extrusion6" add sketch "Skizze7" along normal blind 7 contours L8 L9 L10 L11
sketch "Skizze8" plane through (-0.92, -4.19, -3.12) normal (0, 0, -1) x (-1, 0, 0)
  line L0 (0, 0) -> (0.7, 0) construction
  line L1 (0, 0) -> (0, -1.46) construction
  line L2 (0.7, -1.46) -> (0, -1.46) construction
  line L3 (0.7, 0) -> (0.7, -1.46) construction
  line L4 (0.7, -1.46) -> (0, -1.46)
  line L5 (0, -1.46) -> (0, -0.76)
  line L6 (0, -0.76) -> (0.7, -0.76)
  line L7 (0.7, -0.76) -> (0.7, -1.46)
  point P0 (-0.92, 4.19)
  constraints: 8 end point, 2 parallel, 2 perpendicular, 1 horizontal, 1 point on line
extrude "Extrusion7" add sketch "Skizze8" against normal blind 8
chamfer "Fase2" distance 0.254 angle 45 2 edges at (-1.27, -4.95, -2.42) (-1.27, -5.65, -3.12)
chamfer "Fase3" distance 0.2 angle 45 8 edges at (-0.92, -5.3, 4.88) (-1.27, -5.65, 4.88) (-1.62, -5.3, 4.88) (-1.27, -4.95, 4.88) (-0.92, 1.35, -2.77) (-1.27, 1.35, -3.12) (-1.62, 1.35, -2.77) (-1.27, 1.35, -2.42)
mirror "Spiegeln2" about plane through (0, 0, 0) normal (1, 0, 0) of "Extrusion5", "Fase1"
mirror "Spiegeln3" about plane through (0, 0, 0) normal (1, 0, 0) of "Extrusion6", "Extrusion7", "Fase2", "Fase3"
equation "\"d3\" = d2"
equation "\"d7\" = d0 - d2"
equation "\"d16\" = -0.5 * d13 + 0.5 * d15"
equation "\"d17\" = d16"
equation "\"d31\" = d23"
